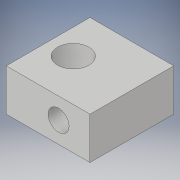
# Autodesk Inventor part: AxleToRodAdapter
Saved by Autodesk Inventor 2017 (Build 210142000, 142)
## iProperties
Created: 2019-01-31
Part Number: AxleToRodAdapter
Material: Generic
Document SubType Name: Modeling
Designer: S338674153
Density: 1 g/cm^3
Appearance: Default
Author: S338674153
Autodesk Inventor part; units mm, degrees
ref_plane "YZ Plane" through (0, 0, 0) normal (1, 0, 0) x (0, 1, 0)
ref_plane "XZ Plane" through (0, 0, 0) normal (0, 1, 0) x (-1, 0, 0)
ref_plane "XY Plane" through (0, 0, 0) normal (0, 0, 1) x (1, 0, 0)
sketch "Sketch1" plane through (0, 0, 0) normal (0, 1, 0) x (-1, 0, 0)
  line L0 (0, 0) -> (50.8, 0)
  line L1 (50.8, 0) -> (50.8, -50.8)
  line L2 (50.8, -50.8) -> (0, -50.8)
  line L3 (0, -50.8) -> (0, 0)
  dimension "d0" = 50.8
  dimension "d1" = 50.8
  constraints: 8 end point, 2 parallel, 1 horizontal, 1 perpendicular
  measures "d0" distance of L1.end L2.end
  measures "d1" distance of L0.end L1.end
extrude "Extrusion1" add sketch "Sketch1" along normal blind 25.4
sketch "Sketch2" plane through (-50.8, 0, 0) normal (0, 0, 1) x (1, 0, 0)
  line L0 (50.8, 0) -> (0, 0) construction
  line L1 (50.8, 0) -> (31.75, 0) construction
  line L2 (31.75, 0) -> (31.75, 12.7) construction
  line L3 (31.75, 12.7) -> (50.8, 12.7) construction
  line L4 (50.8, 12.7) -> (50.8, 0) construction
  circle A0 centre (31.75, 12.7) radius 6.35
  dimension "d4" = 19.05
  dimension "d5" = 12.7
  dimension "d6" = 12.7
  constraints: 8 end point, 2 parallel, 1 centre point, 1 coincident, 1 horizontal, 1 perpendicular
  measures "d4" distance of L2.end L3.end
  measures "d5" distance of L1.end L2.end
  measures "d6" diameter of A0
extrude "Extrusion2" cut sketch "Sketch2" against normal blind 66.675
sketch "Sketch3" plane through (0, 25.4, 0) normal (0, 1, 0) x (1, 0, 0)
  line L0 (-50.8, 0) -> (-35.56, 0) construction
  line L1 (-35.56, 0) -> (-35.56, 25.4) construction
  line L2 (-35.56, 25.4) -> (-50.8, 25.4) construction
  line L3 (-50.8, 25.4) -> (-50.8, 0) construction
  circle A0 centre (-35.56, 25.4) radius 9.525
  point P0 (0, 0)
  dimension "d9" = 15.24
  dimension "d10" = 25.4
  dimension "d11" = 19.05
  constraints: 8 end point, 2 parallel, 1 centre point, 1 coincident, 1 horizontal, 1 perpendicular
  measures "d9" distance of L2.end L1.end
  measures "d10" distance of L1.end L0.end
  measures "d11" diameter of A0
extrude "Extrusion3" cut sketch "Sketch3" against normal blind 31.75
body "Solid1"
